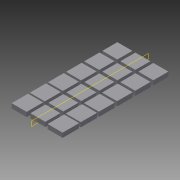
# Autodesk Inventor part: Calibration
Saved by Autodesk Inventor 2013 (Build 170138000, 138)
## iProperties
Created: 2013-02-10
Part Number: Calibration
Material: Generic
Document SubType Name: Modeling
Designer: rhys
Density: 1 g/cm^3
Author: rhys
Autodesk Inventor part; units mm, degrees
ref_plane "YZ Plane" through (0, 0, 0) normal (1, 0, 0) x (0, 1, 0)
ref_plane "XZ Plane" through (0, 0, 0) normal (0, 1, 0) x (-1, 0, 0)
ref_plane "XY Plane" through (0, 0, 0) normal (0, 0, 1) x (1, 0, 0)
sketch "Sketch1" plane through (0, 0, 0) normal (0, 0, 1) x (1, 0, 0)
  line L0 (5, -5) -> (-5, -5)
  line L1 (-5, -5) -> (-5, 5)
  line L2 (-5, 5) -> (5, 5)
  line L3 (5, 5) -> (5, -5)
  line L4 (5, -5) -> (-5, 5) construction
  line L5 (-5, -5) -> (5, 5) construction
  point P0 (0, 0)
  dimension "d0" = 10
  dimension "d2" = 10
  constraints: 12 end point, 2 midpoint, 2 parallel, 1 horizontal, 1 perpendicular
  measures "d0" distance of L1.end L2.end
  measures "d2" distance of L2.end L0.start
extrude "Extrusion1" add sketch "Sketch1" along normal blind 3
pattern_linear "Rectangular Pattern1" count 6 spacing 12 along (0, -1, 0) of "Extrusion1"
sketch "Sketch2" plane through (0, 0, 3) normal (0, 0, 1) x (-1, 0, 0)
  line L0 (-17, -5) -> (-7, -5)
  line L1 (-7, -5) -> (-7, 5)
  line L2 (-7, 5) -> (-17, 5)
  line L3 (-17, 5) -> (-17, -5)
  line L4 (-17, -5) -> (-7, 5) construction
  line L5 (-7, -5) -> (-17, 5) construction
  line L6 (5, 17) -> (-5, 17) construction
  line L7 (-5, 17) -> (-5, 7) construction
  line L8 (-5, 7) -> (5, 7) construction
  line L9 (5, 7) -> (5, 17) construction
  line L10 (5, 29) -> (-5, 29) construction
  line L11 (-5, 29) -> (-5, 19) construction
  line L12 (-5, 19) -> (5, 19) construction
  line L13 (5, 19) -> (5, 29) construction
  line L14 (5, 41) -> (-5, 41) construction
  line L15 (-5, 41) -> (-5, 31) construction
  line L16 (-5, 31) -> (5, 31) construction
  line L17 (5, 31) -> (5, 41) construction
  line L18 (5, 53) -> (-5, 53) construction
  line L19 (-5, 53) -> (-5, 43) construction
  line L20 (-5, 43) -> (5, 43) construction
  line L21 (5, 43) -> (5, 53) construction
  line L22 (5, 65) -> (-5, 65) construction
  line L23 (-5, 65) -> (-5, 55) construction
  line L24 (-5, 55) -> (5, 55) construction
  line L25 (5, 55) -> (5, 65) construction
  line L26 (-7, 17.1) -> (-17, 17.1)
  line L27 (-17, 17.1) -> (-17, 6.9)
  line L28 (-17, 6.9) -> (-7, 6.9)
  line L29 (-7, 6.9) -> (-7, 17.1)
  line L30 (-7, 17.1) -> (-17, 6.9) construction
  line L31 (-17, 17.1) -> (-7, 6.9) construction
  line L32 (-7, 29.2) -> (-17, 29.2)
  line L33 (-17, 29.2) -> (-17, 18.8)
  line L34 (-17, 18.8) -> (-7, 18.8)
  line L35 (-7, 18.8) -> (-7, 29.2)
  line L36 (-7, 29.2) -> (-17, 18.8) construction
  line L37 (-17, 29.2) -> (-7, 18.8) construction
  line L38 (-7, 41.3) -> (-17, 41.3)
  line L39 (-17, 41.3) -> (-17, 30.7)
  line L40 (-17, 30.7) -> (-7, 30.7)
  line L41 (-7, 30.7) -> (-7, 41.3)
  line L42 (-7, 41.3) -> (-17, 30.7) construction
  line L43 (-17, 41.3) -> (-7, 30.7) construction
  line L44 (-7, 53.4) -> (-17, 53.4)
  line L45 (-17, 53.4) -> (-17, 42.6)
  line L46 (-17, 42.6) -> (-7, 42.6)
  line L47 (-7, 42.6) -> (-7, 53.4)
  line L48 (-7, 53.4) -> (-17, 42.6) construction
  line L49 (-17, 53.4) -> (-7, 42.6) construction
  line L50 (-7, 65.5) -> (-17, 65.5)
  line L51 (-17, 65.5) -> (-17, 54.5)
  line L52 (-17, 54.5) -> (-7, 54.5)
  line L53 (-7, 54.5) -> (-7, 65.5)
  line L54 (-7, 65.5) -> (-17, 54.5) construction
  line L55 (-17, 65.5) -> (-7, 54.5) construction
  line L56 (-5, 12) -> (4.1191, 12) construction
  line L57 (-5, 24) -> (3.6782, 24) construction
  line L58 (-5, 36) -> (3.6782, 36) construction
  line L59 (-5, 48) -> (0, 48) construction
  line L60 (-5, 60) -> (2.1339, 60) construction
  point P0 (0, 0)
  point P1 (-12, 0)
  dimension "d8" = 12
  dimension "d10" = 10
  dimension "d11" = 10
  dimension "d12" = 10.2
  dimension "d13" = 5.1
  dimension "d14" = 10.4
  dimension "d15" = 5.2
  dimension "d16" = 5.3
  dimension "d17" = 5.4
  dimension "d18" = 10.6
  dimension "d19" = 10.8
  dimension "d20" = 11
  dimension "d21" = 5.5
  constraints: 82 end point, 16 parallel, 10 collinear, 7 midpoint, 7 perpendicular, 6 horizontal
  measures "d8" distance of point (-12, 0) point (0, 0)
  measures "d10" distance of L0.start L0.end
  measures "d11" distance of L2.end L0.start
  measures "d12" distance of L26.end L27.end
  measures "d13" distance between parallel lines of L56 L28
  measures "d14" distance of L32.end L33.end
  measures "d15" distance between parallel lines of L32 L57
  measures "d16" distance between parallel lines of L58 L40
  measures "d17" distance between parallel lines of L59 L46
  measures "d18" distance of L38.end L39.end
  measures "d19" distance of L44.end L45.end
  measures "d20" distance of L50.end L51.end
  measures "d21" distance between parallel lines of L60 L50
extrude "Extrusion2" add sketch "Sketch2" against normal blind 3
ref_plane "Work Plane1" through (0, -5, 0) normal (1, 0, 0) x (0, 1, 0)
mirror "Mirror1" about plane through (0, -5, 0) normal (1, 0, 0) of "Extrusion2"
body "Solid1"
